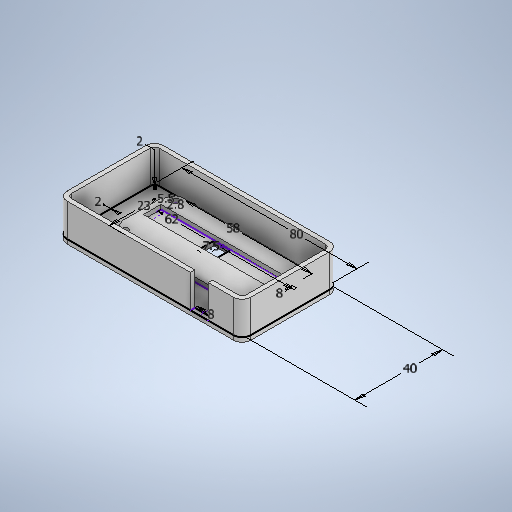
# Autodesk Inventor part: RemoteCasing
Saved by Autodesk Inventor 2025 (Build 290162000, 162)
## iProperties
Created: 2025-02-27
Part Number: RemoteCasing
Material: Generic
Document SubType Name: Modeling
Designer: tvoko
Density: 1 g/cm^3
Appearance: Default
Author: tvoko
Autodesk Inventor part; units mm, degrees
ref_plane "YZ Plane" through (0, 0, 0) normal (1, 0, 0) x (0, 1, 0)
ref_plane "XZ Plane" through (0, 0, 0) normal (0, 1, 0) x (-1, 0, 0)
ref_plane "XY Plane" through (0, 0, 0) normal (0, 0, 1) x (1, 0, 0)
sketch "Sketch1" plane through (0, 0, 0) normal (0, 1, 0) x (-1, 0, 0)
  line L0 (-2, 0) -> (-78, 0)
  line L1 (-80, -2) -> (-80, -38)
  line L2 (-78, -40) -> (-2, -40)
  line L3 (0, -38) -> (0, -2)
  arc A0 (-2, -40) -> (0, -38) centre (-2, -38) ccw
  arc A1 (-80, -38) -> (-78, -40) centre (-78, -38) ccw
  arc A2 (-78, 0) -> (-80, -2) centre (-78, -2) ccw
  arc A3 (0, -2) -> (-2, 0) centre (-2, -2) ccw
  line L4 (2, -2) -> (2, -38)
  arc A4 (-2, -42) -> (2, -38) centre (-2, -38) ccw
  line L5 (-2, -42) -> (-78, -42)
  arc A5 (-82, -38) -> (-78, -42) centre (-78, -38) ccw
  line L6 (-82, -38) -> (-82, -2)
  arc A6 (-78, 2) -> (-82, -2) centre (-78, -2) ccw
  line L7 (-78, 2) -> (-2, 2)
  arc A7 (2, -2) -> (-2, 2) centre (-2, -2) ccw
  line L8 (-13.7168, -12.923) -> (-71.7168, -12.923) construction
  line L9 (-71.7168, -12.923) -> (-71.7168, -35.923) construction
  line L10 (-71.7168, -35.923) -> (-13.7168, -35.923) construction
  line L11 (-13.7168, -35.923) -> (-13.7168, -12.923) construction
  circle A8 centre (-13.7168, -35.923) radius 1.4
  circle A9 centre (-71.7168, -35.923) radius 1.4
  circle A10 centre (-71.7168, -12.923) radius 1.4
  circle A11 centre (-13.7168, -12.923) radius 1.4
  circle A12 centre (-13.7168, -35.923) radius 2.75
  circle A13 centre (-71.7168, -35.923) radius 2.75
  circle A14 centre (-71.7168, -12.923) radius 2.75
  circle A15 centre (-13.7168, -12.923) radius 2.75
  line L12 (-10.9668, -35.923) -> (-10.9668, -12.923) construction
  line L13 (-13.7168, -10.173) -> (-71.7168, -10.173)
  line L14 (-74.4668, -12.923) -> (-74.4668, -35.923) construction
  line L15 (-71.7168, -38.673) -> (-13.7168, -38.673)
  line L16 (-11.7342, -31.1266) -> (-73.7342, -31.1266)
  line L17 (-73.7342, -31.1266) -> (-73.7342, -23.1266)
  line L18 (-73.7342, -23.1266) -> (-11.7342, -23.1266)
  line L19 (-11.7342, -23.1266) -> (-11.7342, -31.1266)
  line L20 (-13.7168, -33.173) -> (-71.7168, -33.173) construction
  line L21 (-13.7168, -15.673) -> (-71.7168, -15.673) construction
  line L22 (-36.25, -30.8183) -> (-43.75, -30.8183)
  line L23 (-43.75, -30.8183) -> (-43.75, -23.3183)
  line L24 (-43.75, -23.3183) -> (-36.25, -23.3183)
  line L25 (-36.25, -23.3183) -> (-36.25, -30.8183)
  line L26 (-40, -40) -> (-40, 0) construction
  line L27 (-62.4106, 2) -> (-62.4106, -6.9509) construction
  line L28 (-58.4106, 0) -> (-66.4106, 0)
  line L29 (-66.4106, 0) -> (-66.4106, 2)
  line L30 (-66.4106, 2) -> (-58.4106, 2)
  line L31 (-58.4106, 2) -> (-58.4106, 0)
  line L32 (-9.3279, -16.0104) -> (-9.3279, -32.8356)
  line L33 (-9.3279, -32.8356) -> (-11.2054, -37.0435)
  line L34 (-9.3279, -16.0104) -> (-11.2054, -11.8025)
  line L35 (-74.1979, -11.7369) -> (-76.2409, -16.0104)
  line L36 (-76.2409, -16.0104) -> (-76.2409, -32.8356)
  line L37 (-76.2409, -32.8356) -> (-74.1979, -37.1091)
  line L38 (-9.3279, -24.423) -> (-76.2409, -24.423) construction
  point P0 (0, 0)
  point P1 (-80, -40)
  point P2 (-80, 0)
  point P3 (0, -40)
  point P4 (-40, -30.8183)
  point P5 (-62.4106, 0)
  point P6 (-10.9668, -24.423)
  dimension "d0" = 40
  dimension "d1" = 80
  dimension "d2" = 2
  dimension "d3" = 2
  dimension "d4" = 2.8
  dimension "d5" = 58
  dimension "d6" = 23
  dimension "d7" = 5.5
  dimension "d8" = 62
  dimension "d9" = 8
  dimension "d10" = 7.5
  dimension "d17" = 8
  constraints: 78 end point, 32 point on circle, 20 tangent, 19 point on line, 16 centre point, 12 parallel, 9 equal radius, 8 coincident, 8 midpoint, 7 perpendicular, 6 horizontal, 3 vertical, 2 equal length, 7 other
  measures "d0" distance of point (-80, 0) point (-80, -40)
  measures "d1" distance of point (-80, -40) point (0, -40)
  measures "d2" radius of A0
  measures "d3" distance between parallel lines of L3 L4
  measures "d4" diameter of A8
  measures "d5" distance of L9.end L10.end
  measures "d6" distance of L10.end L8.start
  measures "d7" diameter of A12
  measures "d8" distance of L16.start L16.end
  measures "d9" distance of L16.end L17.end
  measures "d10" distance of L24.end L22.start
  measures "d17" distance between parallel lines of L29 L31
extrude "Extrusion1" add sketch "Sketch1" against normal blind 2 contours A3 L3 A0 L2 A1 L1 A2 L0 | L0 L31 L7 A7 L4 A4 L5 A5 L6 A6 L29 A2 L1 A1 L2 A0 L3 A3 | L0 L29 L7 L31 | A8 | A9 | A10 | A11 | A12 | A12 L15 A13 L37 L36 L35 A14 L13 A15 L34 L32 L33 | A13 | A15 | A14 | L16 L17 L18 L19
extrude "Extrusion2" add sketch "Sketch1" along normal blind 15 contours L0 L31 L7 A7 L4 A4 L5 A5 L6 A6 L29 A2 L1 A1 L2 A0 L3 A3
extrude "Extrusion3" add sketch "Sketch1" along normal blind 2 contours A12 | A12 L15 A13 L37 L36 L35 A14 L13 A15 L34 L32 L33 | A13 | A15 | A14
body "Solid1"
